Autodesk Fusion 360 part; units mm, degrees
(part 8 of 18)
  line L5222 (108.6972, -31.4557) -> (122.6972, -31.4557)
  line L5223 (122.6972, -45.4557) -> (108.6972, -45.4557)
  line L5224 (108.6972, -45.4557) -> (108.6972, -31.4557)
  line L5225 (89.6472, -26.4057) -> (89.6472, -12.4056)
  line L5226 (103.6472, -12.4056) -> (103.6472, -26.4057)
  line L5227 (103.6472, -26.4057) -> (89.6472, -26.4057)
  line L5228 (89.6472, -12.4056) -> (103.6472, -12.4056)
  line L5229 (89.6472, -31.4557) -> (103.6472, -31.4557)
  line L5230 (103.6472, -31.4557) -> (103.6472, -45.4557)
  line L5231 (103.6472, -45.4557) -> (89.6472, -45.4557)
  line L5232 (89.6472, -45.4557) -> (89.6472, -31.4557)
  line L5233 (89.6472, -69.5811) -> (103.6472, -69.5811)
  line L5234 (103.6472, -83.5812) -> (89.6472, -83.5812)
  line L5235 (103.6472, -69.5811) -> (103.6472, -83.5812)
  line L5236 (89.6472, -83.5812) -> (89.6472, -69.5811)
  line L5237 (89.6472, -64.5184) -> (89.6472, -50.5184)
  line L5238 (103.6472, -64.5184) -> (89.6472, -64.5184)
  line L5239 (89.6472, -50.5184) -> (103.6472, -50.5184)
  line L5240 (103.6472, -50.5184) -> (103.6472, -64.5184)
  line L5241 (184.8974, -83.5812) -> (184.8974, -69.5811)
  line L5242 (198.8974, -83.5812) -> (184.8974, -83.5812)
  line L5243 (198.8974, -69.5811) -> (198.8974, -83.5812)
  line L5244 (184.8974, -69.5811) -> (198.8974, -69.5811)
  line L5245 (184.8974, -12.4056) -> (198.8974, -12.4056)
  line L5246 (198.8974, -12.4056) -> (198.8974, -26.4057)
  line L5247 (198.8974, -26.4057) -> (184.8974, -26.4057)
  line L5248 (184.8974, -26.4057) -> (184.8974, -12.4056)
  line L5249 (84.5972, -83.5812) -> (70.5971, -83.5812)
  line L5250 (70.5971, -69.5811) -> (84.5972, -69.5811)
  line L5251 (70.5971, -83.5812) -> (70.5971, -69.5811)
  line L5252 (84.5972, -69.5811) -> (84.5972, -83.5812)
  line L5253 (70.5971, -31.4557) -> (84.5972, -31.4557)
  line L5254 (70.5971, -45.4557) -> (70.5971, -31.4557)
  line L5255 (84.5972, -31.4557) -> (84.5972, -45.4557)
  line L5256 (84.5972, -45.4557) -> (70.5971, -45.4557)
  line L5257 (70.5971, -12.4056) -> (84.5972, -12.4056)
  line L5258 (84.5972, -12.4056) -> (84.5972, -26.4057)
  line L5259 (70.5971, -26.4057) -> (70.5971, -12.4056)
  line L5260 (84.5972, -26.4057) -> (70.5971, -26.4057)
  line L5261 (70.5971, -50.5184) -> (84.5972, -50.5184)
  line L5262 (84.5972, -64.5184) -> (70.5971, -64.5184)
  line L5263 (70.5971, -64.5184) -> (70.5971, -50.5184)
  line L5264 (84.5972, -50.5184) -> (84.5972, -64.5184)
  line L5265 (65.5471, -83.5812) -> (51.5471, -83.5812)
  line L5266 (51.5471, -69.5811) -> (65.5471, -69.5811)
  line L5267 (51.5471, -83.5812) -> (51.5471, -69.5811)
  line L5268 (65.5471, -69.5811) -> (65.5471, -83.5812)
  line L5269 (65.5471, -50.5184) -> (65.5471, -64.5184)
  line L5270 (51.5471, -64.5184) -> (51.5471, -50.5184)
  line L5271 (65.5471, -64.5184) -> (51.5471, -64.5184)
  line L5272 (51.5471, -50.5184) -> (65.5471, -50.5184)
  line L5273 (51.5471, -45.4557) -> (51.5471, -31.4557)
  line L5274 (65.5471, -31.4557) -> (65.5471, -45.4557)
  line L5275 (51.5471, -31.4557) -> (65.5471, -31.4557)
  line L5276 (65.5471, -45.4557) -> (51.5471, -45.4557)
  line L5277 (46.4971, -64.5184) -> (32.4971, -64.5184)
  line L5278 (32.4971, -64.5184) -> (32.4971, -50.5184)
  line L5279 (32.4971, -50.5184) -> (46.4971, -50.5184)
  line L5280 (46.4971, -50.5184) -> (46.4971, -64.5184)
  line L5281 (32.4971, -69.5811) -> (46.4971, -69.5811)
  line L5282 (32.4971, -83.5812) -> (32.4971, -69.5811)
  line L5283 (46.4971, -83.5812) -> (32.4971, -83.5812)
  line L5284 (46.4971, -69.5811) -> (46.4971, -83.5812)
  line L5285 (13.447, -69.5811) -> (27.4471, -69.5811)
  line L5286 (27.4471, -83.5812) -> (13.447, -83.5812)
  line L5287 (27.4471, -69.5811) -> (27.4471, -83.5812)
  line L5288 (13.447, -83.5812) -> (13.447, -69.5811)
  line L5289 (-5.603, -69.5811) -> (8.397, -69.5811)
  line L5290 (8.397, -83.5812) -> (-5.603, -83.5812)
  line L5291 (8.397, -69.5811) -> (8.397, -83.5812)
  line L5292 (-5.603, -83.5812) -> (-5.603, -69.5811)
  line L5293 (65.5471, -12.4056) -> (65.5471, -26.4057)
  line L5294 (51.5471, -12.4056) -> (65.5471, -12.4056)
  line L5295 (51.5471, -26.4057) -> (51.5471, -12.4056)
  line L5296 (65.5471, -26.4057) -> (51.5471, -26.4057)
  line L5297 (32.4971, -31.4557) -> (46.4971, -31.4557)
  line L5298 (46.4971, -45.4557) -> (32.4971, -45.4557)
  line L5299 (32.4971, -45.4557) -> (32.4971, -31.4557)
  line L5300 (46.4971, -31.4557) -> (46.4971, -45.4557)
  line L5301 (46.4971, -12.4056) -> (46.4971, -26.4057)
  line L5302 (32.4971, -12.4056) -> (46.4971, -12.4056)
  line L5303 (32.4971, -26.4057) -> (32.4971, -12.4056)
  line L5304 (46.4971, -26.4057) -> (32.4971, -26.4057)
  line L5305 (13.447, -26.4057) -> (13.447, -12.4056)
  line L5306 (27.4471, -26.4057) -> (13.447, -26.4057)
  line L5307 (27.4471, -12.4056) -> (27.4471, -26.4057)
  line L5308 (13.447, -12.4056) -> (27.4471, -12.4056)
  line L5309 (13.447, -64.5184) -> (13.447, -50.5184)
  line L5310 (27.4471, -64.5184) -> (13.447, -64.5184)
  line L5311 (13.447, -50.5184) -> (27.4471, -50.5184)
  line L5312 (27.4471, -50.5184) -> (27.4471, -64.5184)
  line L5313 (13.447, -31.4557) -> (27.4471, -31.4557)
  line L5314 (27.4471, -45.4557) -> (13.447, -45.4557)
  line L5315 (27.4471, -31.4557) -> (27.4471, -45.4557)
  line L5316 (13.447, -45.4557) -> (13.447, -31.4557)
  line L5317 (8.397, -12.4056) -> (8.397, -26.4057)
  line L5318 (-5.603, -12.4056) -> (8.397, -12.4056)
  line L5319 (-5.603, -26.4057) -> (-5.603, -12.4056)
  line L5320 (8.397, -26.4057) -> (-5.603, -26.4057)
  line L5321 (8.397, -45.4557) -> (-5.603, -45.4557)
  line L5322 (8.397, -31.4557) -> (8.397, -45.4557)
  line L5323 (-5.603, -45.4557) -> (-5.603, -31.4557)
  line L5324 (-5.603, -31.4557) -> (8.397, -31.4557)
  line L5325 (-5.603, -50.5184) -> (8.397, -50.5184)
  line L5326 (8.397, -50.5184) -> (8.397, -64.5184)
  line L5327 (-5.603, -64.5184) -> (-5.603, -50.5184)
  line L5328 (8.397, -64.5184) -> (-5.603, -64.5184)
  line L5329 (217.9474, -50.5184) -> (217.9474, -64.5184)
  line L5330 (203.9474, -50.5184) -> (217.9474, -50.5184)
  line L5331 (217.9474, -64.5184) -> (203.9474, -64.5184)
  line L5332 (203.9474, -64.5184) -> (203.9474, -50.5184)
  line L5333 (203.9474, -31.4557) -> (217.9474, -31.4557)
  line L5334 (217.9474, -45.4557) -> (203.9474, -45.4557)
  line L5335 (203.9474, -45.4557) -> (203.9474, -31.4557)
  line L5336 (217.9474, -31.4557) -> (217.9474, -45.4557)
  line L5337 (217.9474, -12.4056) -> (217.9474, -26.4057)
  line L5338 (203.9474, -26.4057) -> (203.9474, -12.4056)
  line L5339 (217.9474, -26.4057) -> (203.9474, -26.4057)
  line L5340 (203.9474, -12.4056) -> (217.9474, -12.4056)
  line L5341 (203.9474, -69.5811) -> (217.9474, -69.5811)
  line L5342 (203.9474, -83.5812) -> (203.9474, -69.5811)
  line L5343 (217.9474, -83.5812) -> (203.9474, -83.5812)
  line L5344 (217.9474, -69.5811) -> (217.9474, -83.5812)
  line L5345 (184.8974, -45.4557) -> (184.8974, -31.4557)
  line L5346 (198.8974, -31.4557) -> (198.8974, -45.4557)
  line L5347 (184.8974, -31.4557) -> (198.8974, -31.4557)
  line L5348 (198.8974, -45.4557) -> (184.8974, -45.4557)
  line L5349 (177.1674, -3.048) -> (172.3373, -3.048)
  line L5350 (177.1674, -5.588) -> (177.1674, -3.048)
  line L5351 (177.1674, -5.588) -> (172.3373, -5.588)
  line L5352 (172.3373, -5.588) -> (172.3373, -3.048)
  line L5353 (188.5494, -4.29) -> (189.1994, -4.29)
  line L5354 (188.5494, -5.49) -> (188.5494, -4.29)
  line L5355 (189.1994, -4.29) -> (189.1994, -5.49)
  line L5356 (189.1994, -5.49) -> (188.5494, -5.49)
  line L5357 (188.3993, -5.49) -> (187.7493, -5.49)
  line L5358 (188.3993, -4.29) -> (188.3993, -5.49)
  line L5359 (187.7493, -4.29) -> (188.3993, -4.29)
  line L5360 (187.7493, -5.49) -> (187.7493, -4.29)
  line L5361 (187.6243, -4.29) -> (187.6243, -5.49)
  line L5362 (187.6243, -5.49) -> (187.2243, -5.49)
  line L5363 (187.2243, -4.29) -> (187.6243, -4.29)
  line L5364 (187.2243, -5.49) -> (187.2243, -4.29)
  line L5365 (187.1242, -5.49) -> (186.7242, -5.49)
  line L5366 (186.7242, -4.29) -> (187.1242, -4.29)
  line L5367 (187.1242, -4.29) -> (187.1242, -5.49)
  line L5368 (186.7242, -5.49) -> (186.7242, -4.29)
  line L5369 (186.2243, -4.29) -> (186.6243, -4.29)
  line L5370 (186.2243, -5.49) -> (186.2243, -4.29)
  line L5371 (186.6243, -5.49) -> (186.2243, -5.49)
  line L5372 (186.6243, -4.29) -> (186.6243, -5.49)
  line L5373 (185.7244, -5.49) -> (185.7244, -4.29)
  line L5374 (186.1244, -4.29) -> (186.1244, -5.49)
  line L5375 (186.1244, -5.49) -> (185.7244, -5.49)
  line L5376 (185.7244, -4.29) -> (186.1244, -4.29)
  line L5377 (185.6243, -5.49) -> (185.2243, -5.49)
  line L5378 (185.2243, -5.49) -> (185.2243, -4.29)
  line L5379 (185.2243, -4.29) -> (185.6243, -4.29)
  line L5380 (185.6243, -4.29) -> (185.6243, -5.49)
  line L5381 (185.1244, -4.29) -> (185.1244, -5.49)
  line L5382 (185.1244, -5.49) -> (184.7244, -5.49)
  line L5383 (184.7244, -4.29) -> (185.1244, -4.29)
  line L5384 (184.7244, -5.49) -> (184.7244, -4.29)
  line L5385 (184.6243, -5.49) -> (184.2243, -5.49)
  line L5386 (184.2243, -4.29) -> (184.6243, -4.29)
  line L5387 (184.6243, -4.29) -> (184.6243, -5.49)
  line L5388 (184.2243, -5.49) -> (184.2243, -4.29)
  line L5389 (184.1242, -5.49) -> (183.7242, -5.49)
  line L5390 (183.7242, -5.49) -> (183.7242, -4.29)
  line L5391 (183.7242, -4.29) -> (184.1242, -4.29)
  line L5392 (184.1242, -4.29) -> (184.1242, -5.49)
  line L5393 (183.5992, -5.49) -> (182.9492, -5.49)
  line L5394 (183.5992, -4.29) -> (183.5992, -5.49)
  line L5395 (182.9492, -4.29) -> (183.5992, -4.29)
  line L5396 (182.9492, -5.49) -> (182.9492, -4.29)
  line L5397 (182.7994, -5.49) -> (182.1493, -5.49)
  line L5398 (182.7994, -4.29) -> (182.7994, -5.49)
  line L5399 (182.1493, -4.29) -> (182.7994, -4.29)
  line L5400 (182.1493, -5.49) -> (182.1493, -4.29)
  line L5401 (189.4747, -3.4901) -> (189.6943, -3.2705)
  line L5402 (190.2943, -3.2705) -> (190.5139, -3.4901)
  line L5403 (190.2943, -5.4097) -> (189.9943, -5.4901)
  line L5404 (190.5139, -3.4901) -> (190.5943, -3.7901)
  line L5405 (189.6943, -5.4097) -> (189.4747, -5.1901)
  line L5406 (189.6943, -3.2705) -> (189.9943, -3.1901)
  line L5407 (190.5139, -5.1901) -> (190.2943, -5.4097)
  line L5408 (189.3943, -3.7901) -> (189.4747, -3.4901)
  line L5409 (189.3943, -4.8901) -> (189.3943, -3.7901)
  line L5410 (189.9943, -5.4901) -> (189.6943, -5.4097)
  line L5411 (189.4747, -5.1901) -> (189.3943, -4.8901)
  line L5412 (189.9943, -3.1901) -> (190.2943, -3.2705)
  line L5413 (190.5943, -4.8901) -> (190.5139, -5.1901)
  line L5414 (190.5943, -3.7901) -> (190.5943, -4.8901)
  line L5415 (181.6545, -5.4097) -> (181.3545, -5.4901)
  line L5416 (181.0545, -5.4097) -> (180.8348, -5.1901)
  line L5417 (180.7544, -3.7901) -> (180.8348, -3.4901)
  line L5418 (181.8741, -3.4901) -> (181.9545, -3.7901)
  line L5419 (180.8348, -5.1901) -> (180.7544, -4.8901)
  line L5420 (181.9545, -3.7901) -> (181.9545, -4.8901)
  line L5421 (181.9545, -4.8901) -> (181.8741, -5.1901)
  line L5422 (181.8741, -5.1901) -> (181.6545, -5.4097)
  line L5423 (180.8348, -3.4901) -> (181.0545, -3.2705)
  line L5424 (181.3545, -3.1901) -> (181.6545, -3.2705)
  line L5425 (181.0545, -3.2705) -> (181.3545, -3.1901)
  line L5426 (180.7544, -4.8901) -> (180.7544, -3.7901)
  line L5427 (181.3545, -5.4901) -> (181.0545, -5.4097)
  line L5428 (181.6545, -3.2705) -> (181.8741, -3.4901)
  line L5429 (189.3943, 0.21) -> (189.4747, 0.51)
  line L5430 (189.3943, -0.59) -> (189.3943, 0.21)
  line L5431 (190.5943, 0.21) -> (190.5943, -0.59)
  line L5432 (190.5139, -0.89) -> (190.2943, -1.1096)
  line L5433 (190.5139, 0.51) -> (190.5943, 0.21)
  line L5434 (189.4747, 0.51) -> (189.6943, 0.7297)
  line L5435 (189.6943, 0.7297) -> (189.9943, 0.81)
  line L5436 (190.5943, -0.59) -> (190.5139, -0.89)
  line L5437 (189.9943, -1.19) -> (189.6943, -1.1096)
  line L5438 (189.9943, 0.81) -> (190.2943, 0.7297)
  line L5439 (190.2943, 0.7297) -> (190.5139, 0.51)
  line L5440 (190.2943, -1.1096) -> (189.9943, -1.19)
  line L5441 (189.6943, -1.1096) -> (189.4747, -0.89)
  line L5442 (189.4747, -0.89) -> (189.3943, -0.59)
  line L5443 (181.0545, 0.7297) -> (181.3545, 0.81)
  line L5444 (181.3545, 0.81) -> (181.6545, 0.7297)
  line L5445 (181.8741, 0.51) -> (181.9545, 0.21)
  line L5446 (180.8348, 0.51) -> (181.0545, 0.7297)
  line L5447 (181.0545, -1.1096) -> (180.8348, -0.89)
  line L5448 (180.8348, -0.89) -> (180.7544, -0.59)
  line L5449 (181.8741, -0.89) -> (181.6545, -1.1096)
  line L5450 (181.9545, 0.21) -> (181.9545, -0.59)
  line L5451 (181.9545, -0.59) -> (181.8741, -0.89)
  line L5452 (180.7544, -0.59) -> (180.7544, 0.21)
  line L5453 (181.6545, -1.1096) -> (181.3545, -1.19)
  line L5454 (180.7544, 0.21) -> (180.8348, 0.51)
  line L5455 (181.6545, 0.7297) -> (181.8741, 0.51)
  line L5456 (181.3545, -1.19) -> (181.0545, -1.1096)
  line L5457 (200.3611, -1.4222) -> (200.3611, -2.3878)
  line L5458 (200.3611, -2.3878) -> (199.453, -2.3878)
  line L5459 (199.453, -1.4222) -> (200.3611, -1.4222)
  line L5460 (199.453, -2.3878) -> (199.453, -1.4222)
  line L5461 (200.9597, -1.4222) -> (201.8678, -1.4222)
  line L5462 (201.8678, -1.4222) -> (201.8678, -2.3878)
  line L5463 (201.8678, -2.3878) -> (200.9597, -2.3878)
  line L5464 (200.9597, -2.3878) -> (200.9597, -1.4222)
  line L5465 (207.2836, -6.3137) -> (207.2836, -6.0121)
  line L5466 (207.2836, -6.0121) -> (208.0502, -6.0121)
  line L5467 (208.0502, -6.0121) -> (208.0502, -6.3137)
  line L5468 (208.0502, -6.3137) -> (207.2836, -6.3137)
  line L5469 (208.0502, -6.4122) -> (208.0502, -6.7138)
  line L5470 (207.2836, -6.7138) -> (207.2836, -6.4122)
  line L5471 (208.0502, -6.7138) -> (207.2836, -6.7138)
  line L5472 (207.2836, -6.4122) -> (208.0502, -6.4122)
  line L5473 (208.0502, -7.1138) -> (207.2836, -7.1138)
  line L5474 (207.2836, -7.1138) -> (207.2836, -6.8122)
  line L5475 (207.2836, -6.8122) -> (208.0502, -6.8122)
  line L5476 (208.0502, -6.8122) -> (208.0502, -7.1138)
  line L5477 (208.0502, -7.212) -> (208.0502, -7.5136)
  line L5478 (207.2836, -7.5136) -> (207.2836, -7.212)
  line L5479 (208.0502, -7.5136) -> (207.2836, -7.5136)
  line L5480 (207.2836, -7.212) -> (208.0502, -7.212)
  line L5481 (207.2836, -7.6121) -> (208.0502, -7.6121)
  line L5482 (208.0502, -7.6121) -> (208.0502, -7.9137)
  line L5483 (208.0502, -7.9137) -> (207.2836, -7.9137)
  line L5484 (207.2836, -7.9137) -> (207.2836, -7.6121)
  line L5485 (207.2836, -8.3137) -> (207.2836, -8.0121)
  line L5486 (208.0502, -8.3137) -> (207.2836, -8.3137)
  line L5487 (207.2836, -8.0121) -> (208.0502, -8.0121)
  line L5488 (208.0502, -8.0121) -> (208.0502, -8.3137)
  line L5489 (208.0502, -8.7138) -> (207.2836, -8.7138)
  line L5490 (208.0502, -8.4122) -> (208.0502, -8.7138)
  line L5491 (207.2836, -8.4122) -> (208.0502, -8.4122)
  line L5492 (207.2836, -8.7138) -> (207.2836, -8.4122)
  line L5493 (208.0502, -8.8122) -> (208.0502, -9.1138)
  line L5494 (208.0502, -9.1138) -> (207.2836, -9.1138)
  line L5495 (207.2836, -8.8122) -> (208.0502, -8.8122)
  line L5496 (207.2836, -9.1138) -> (207.2836, -8.8122)
  line L5497 (208.0502, -9.5136) -> (207.2836, -9.5136)
  line L5498 (208.0502, -9.212) -> (208.0502, -9.5136)
  line L5499 (207.2836, -9.5136) -> (207.2836, -9.212)
  line L5500 (207.2836, -9.212) -> (208.0502, -9.212)
  line L5501 (208.0502, -9.9137) -> (207.2836, -9.9137)
  line L5502 (208.0502, -9.6121) -> (208.0502, -9.9137)
  line L5503 (207.2836, -9.9137) -> (207.2836, -9.6121)
  line L5504 (207.2836, -9.6121) -> (208.0502, -9.6121)
  line L5505 (207.2836, -10.3137) -> (207.2836, -10.0121)
  line L5506 (208.0502, -10.0121) -> (208.0502, -10.3137)
  line L5507 (208.0502, -10.3137) -> (207.2836, -10.3137)
  line L5508 (207.2836, -10.0121) -> (208.0502, -10.0121)
  line L5509 (208.0502, -10.7138) -> (207.2836, -10.7138)
  line L5510 (207.2836, -10.4122) -> (208.0502, -10.4122)
  line L5511 (207.2836, -10.7138) -> (207.2836, -10.4122)
  line L5512 (208.0502, -10.4122) -> (208.0502, -10.7138)
  line L5513 (207.2836, -11.1138) -> (207.2836, -10.8122)
  line L5514 (208.0502, -11.1138) -> (207.2836, -11.1138)
  line L5515 (208.0502, -10.8122) -> (208.0502, -11.1138)
  line L5516 (207.2836, -10.8122) -> (208.0502, -10.8122)
  line L5517 (208.0502, -11.212) -> (208.0502, -11.5136)
  line L5518 (207.2836, -11.5136) -> (207.2836, -11.212)
  line L5519 (207.2836, -11.212) -> (208.0502, -11.212)
  line L5520 (208.0502, -11.5136) -> (207.2836, -11.5136)
  line L5521 (208.6254, -11.7873) -> (208.6254, -12.5539)
  line L5522 (208.6254, -12.5539) -> (208.3238, -12.5539)
  line L5523 (208.3238, -12.5539) -> (208.3238, -11.7873)
  line L5524 (208.3238, -11.7873) -> (208.6254, -11.7873)
  line L5525 (209.0252, -11.7873) -> (209.0252, -12.5539)
  line L5526 (208.7236, -11.7873) -> (209.0252, -11.7873)
  line L5527 (209.0252, -12.5539) -> (208.7236, -12.5539)
  line L5528 (208.7236, -12.5539) -> (208.7236, -11.7873)
  line L5529 (209.4252, -11.7873) -> (209.4252, -12.5539)
  line L5530 (209.1236, -12.5539) -> (209.1236, -11.7873)
  line L5531 (209.4252, -12.5539) -> (209.1236, -12.5539)
  line L5532 (209.1236, -11.7873) -> (209.4252, -11.7873)
  line L5533 (209.5237, -11.7873) -> (209.8253, -11.7873)
  line L5534 (209.8253, -12.5539) -> (209.5237, -12.5539)
  line L5535 (209.5237, -12.5539) -> (209.5237, -11.7873)
  line L5536 (209.8253, -11.7873) -> (209.8253, -12.5539)
  line L5537 (209.9237, -11.7873) -> (210.2253, -11.7873)
  line L5538 (210.2253, -11.7873) -> (210.2253, -12.5539)
  line L5539 (210.2253, -12.5539) -> (209.9237, -12.5539)
  line L5540 (209.9237, -12.5539) -> (209.9237, -11.7873)
  line L5541 (210.3238, -11.7873) -> (210.6254, -11.7873)
  line L5542 (210.6254, -12.5539) -> (210.3238, -12.5539)
  line L5543 (210.6254, -11.7873) -> (210.6254, -12.5539)
  line L5544 (210.3238, -12.5539) -> (210.3238, -11.7873)
  line L5545 (211.0252, -12.5539) -> (210.7236, -12.5539)
  line L5546 (211.0252, -11.7873) -> (211.0252, -12.5539)
  line L5547 (210.7236, -11.7873) -> (211.0252, -11.7873)
  line L5548 (210.7236, -12.5539) -> (210.7236, -11.7873)
  line L5549 (211.1236, -12.5539) -> (211.1236, -11.7873)
  line L5550 (211.4252, -12.5539) -> (211.1236, -12.5539)
  line L5551 (211.1236, -11.7873) -> (211.4252, -11.7873)
  line L5552 (211.4252, -11.7873) -> (211.4252, -12.5539)
  line L5553 (211.5237, -11.7873) -> (211.8253, -11.7873)
  line L5554 (211.5237, -12.5539) -> (211.5237, -11.7873)
  line L5555 (211.8253, -12.5539) -> (211.5237, -12.5539)
  line L5556 (211.8253, -11.7873) -> (211.8253, -12.5539)
  line L5557 (211.9237, -12.5539) -> (211.9237, -11.7873)
  line L5558 (212.2253, -12.5539) -> (211.9237, -12.5539)
  line L5559 (212.2253, -11.7873) -> (212.2253, -12.5539)
  line L5560 (211.9237, -11.7873) -> (212.2253, -11.7873)
  line L5561 (212.3238, -12.5539) -> (212.3238, -11.7873)
  line L5562 (212.3238, -11.7873) -> (212.6254, -11.7873)
  line L5563 (212.6254, -12.5539) -> (212.3238, -12.5539)
  line L5564 (212.6254, -11.7873) -> (212.6254, -12.5539)
  line L5565 (213.0252, -11.7873) -> (213.0252, -12.5539)
  line L5566 (212.7236, -12.5539) -> (212.7236, -11.7873)
  line L5567 (213.0252, -12.5539) -> (212.7236, -12.5539)
  line L5568 (212.7236, -11.7873) -> (213.0252, -11.7873)
  line L5569 (213.1236, -12.5539) -> (213.1236, -11.7873)
  line L5570 (213.4252, -11.7873) -> (213.4252, -12.5539)
  line L5571 (213.4252, -12.5539) -> (213.1236, -12.5539)
  line L5572 (213.1236, -11.7873) -> (213.4252, -11.7873)
  line L5573 (213.5237, -12.5539) -> (213.5237, -11.7873)
  line L5574 (213.8253, -12.5539) -> (213.5237, -12.5539)
  line L5575 (213.8253, -11.7873) -> (213.8253, -12.5539)
  line L5576 (213.5237, -11.7873) -> (213.8253, -11.7873)
  line L5577 (214.8653, -11.212) -> (214.8653, -11.5136)
  line L5578 (214.0987, -11.212) -> (214.8653, -11.212)
  line L5579 (214.8653, -11.5136) -> (214.0987, -11.5136)
  line L5580 (214.0987, -11.5136) -> (214.0987, -11.212)
  line L5581 (214.0987, -11.1138) -> (214.0987, -10.8122)
  line L5582 (214.8653, -11.1138) -> (214.0987, -11.1138)
  line L5583 (214.0987, -10.8122) -> (214.8653, -10.8122)
  line L5584 (214.8653, -10.8122) -> (214.8653, -11.1138)
  line L5585 (214.0987, -10.7138) -> (214.0987, -10.4122)
  line L5586 (214.0987, -10.4122) -> (214.8653, -10.4122)
  line L5587 (214.8653, -10.4122) -> (214.8653, -10.7138)
  line L5588 (214.8653, -10.7138) -> (214.0987, -10.7138)
  line L5589 (214.0987, -10.0121) -> (214.8653, -10.0121)
  line L5590 (214.8653, -10.0121) -> (214.8653, -10.3137)
  line L5591 (214.8653, -10.3137) -> (214.0987, -10.3137)
  line L5592 (214.0987, -10.3137) -> (214.0987, -10.0121)
  line L5593 (214.8653, -9.6121) -> (214.8653, -9.9137)
  line L5594 (214.0987, -9.6121) -> (214.8653, -9.6121)
  line L5595 (214.8653, -9.9137) -> (214.0987, -9.9137)
  line L5596 (214.0987, -9.9137) -> (214.0987, -9.6121)
  line L5597 (214.0987, -9.212) -> (214.8653, -9.212)
  line L5598 (214.8653, -9.212) -> (214.8653, -9.5136)
  line L5599 (214.0987, -9.5136) -> (214.0987, -9.212)
  line L5600 (214.8653, -9.5136) -> (214.0987, -9.5136)
  line L5601 (214.0987, -9.1138) -> (214.0987, -8.8122)
  line L5602 (214.0987, -8.8122) -> (214.8653, -8.8122)
  line L5603 (214.8653, -9.1138) -> (214.0987, -9.1138)
  line L5604 (214.8653, -8.8122) -> (214.8653, -9.1138)
  line L5605 (214.0987, -8.7138) -> (214.0987, -8.4122)
  line L5606 (214.8653, -8.4122) -> (214.8653, -8.7138)
  line L5607 (214.0987, -8.4122) -> (214.8653, -8.4122)
  line L5608 (214.8653, -8.7138) -> (214.0987, -8.7138)
  line L5609 (214.8653, -8.0121) -> (214.8653, -8.3137)
  line L5610 (214.0987, -8.3137) -> (214.0987, -8.0121)
  line L5611 (214.0987, -8.0121) -> (214.8653, -8.0121)
  line L5612 (214.8653, -8.3137) -> (214.0987, -8.3137)
  line L5613 (214.8653, -7.9137) -> (214.0987, -7.9137)
  line L5614 (214.0987, -7.9137) -> (214.0987, -7.6121)
  line L5615 (214.0987, -7.6121) -> (214.8653, -7.6121)
  line L5616 (214.8653, -7.6121) -> (214.8653, -7.9137)
  line L5617 (214.8653, -7.212) -> (214.8653, -7.5136)
  line L5618 (214.0987, -7.212) -> (214.8653, -7.212)
  line L5619 (214.0987, -7.5136) -> (214.0987, -7.212)
  line L5620 (214.8653, -7.5136) -> (214.0987, -7.5136)
  line L5621 (214.8653, -7.1138) -> (214.0987, -7.1138)
  line L5622 (214.0987, -7.1138) -> (214.0987, -6.8122)
  line L5623 (214.8653, -6.8122) -> (214.8653, -7.1138)
  line L5624 (214.0987, -6.8122) -> (214.8653, -6.8122)
  line L5625 (214.8653, -6.4122) -> (214.8653, -6.7138)
  line L5626 (214.0987, -6.7138) -> (214.0987, -6.4122)
  line L5627 (214.0987, -6.4122) -> (214.8653, -6.4122)
  line L5628 (214.8653, -6.7138) -> (214.0987, -6.7138)
  line L5629 (214.8653, -6.0121) -> (214.8653, -6.3137)
  line L5630 (214.8653, -6.3137) -> (214.0987, -6.3137)
  line L5631 (214.0987, -6.3137) -> (214.0987, -6.0121)
  line L5632 (214.0987, -6.0121) -> (214.8653, -6.0121)
  line L5633 (213.8253, -5.7388) -> (213.5237, -5.7388)
  line L5634 (213.5237, -4.9722) -> (213.8253, -4.9722)
  line L5635 (213.8253, -4.9722) -> (213.8253, -5.7388)
  line L5636 (213.5237, -5.7388) -> (213.5237, -4.9722)
  line L5637 (213.1236, -4.9722) -> (213.4252, -4.9722)
  line L5638 (213.1236, -5.7388) -> (213.1236, -4.9722)
  line L5639 (213.4252, -4.9722) -> (213.4252, -5.7388)
  line L5640 (213.4252, -5.7388) -> (213.1236, -5.7388)
  line L5641 (212.7236, -5.7388) -> (212.7236, -4.9722)
  line L5642 (212.7236, -4.9722) -> (213.0252, -4.9722)
  line L5643 (213.0252, -5.7388) -> (212.7236, -5.7388)
  line L5644 (213.0252, -4.9722) -> (213.0252, -5.7388)
  line L5645 (212.6254, -4.9722) -> (212.6254, -5.7388)
  line L5646 (212.3238, -4.9722) -> (212.6254, -4.9722)
  line L5647 (212.6254, -5.7388) -> (212.3238, -5.7388)
  line L5648 (212.3238, -5.7388) -> (212.3238, -4.9722)
  line L5649 (212.2253, -5.7388) -> (211.9237, -5.7388)
  line L5650 (211.9237, -4.9722) -> (212.2253, -4.9722)
  line L5651 (212.2253, -4.9722) -> (212.2253, -5.7388)
  line L5652 (211.9237, -5.7388) -> (211.9237, -4.9722)
  line L5653 (211.5237, -5.7388) -> (211.5237, -4.9722)
  line L5654 (211.5237, -4.9722) -> (211.8253, -4.9722)
  line L5655 (211.8253, -5.7388) -> (211.5237, -5.7388)
  line L5656 (211.8253, -4.9722) -> (211.8253, -5.7388)
  line L5657 (211.4252, -4.9722) -> (211.4252, -5.7388)
  line L5658 (211.1236, -5.7388) -> (211.1236, -4.9722)
  line L5659 (211.1236, -4.9722) -> (211.4252, -4.9722)
  line L5660 (211.4252, -5.7388) -> (211.1236, -5.7388)
  line L5661 (211.0252, -4.9722) -> (211.0252, -5.7388)
  line L5662 (210.7236, -4.9722) -> (211.0252, -4.9722)
  line L5663 (210.7236, -5.7388) -> (210.7236, -4.9722)
  line L5664 (211.0252, -5.7388) -> (210.7236, -5.7388)
  line L5665 (210.6254, -4.9722) -> (210.6254, -5.7388)
  line L5666 (210.3238, -4.9722) -> (210.6254, -4.9722)
  line L5667 (210.6254, -5.7388) -> (210.3238, -5.7388)
  line L5668 (210.3238, -5.7388) -> (210.3238, -4.9722)
  line L5669 (209.9237, -5.7388) -> (209.9237, -4.9722)
  line L5670 (210.2253, -4.9722) -> (210.2253, -5.7388)
  line L5671 (209.9237, -4.9722) -> (210.2253, -4.9722)
  line L5672 (210.2253, -5.7388) -> (209.9237, -5.7388)
  line L5673 (209.8253, -5.7388) -> (209.5237, -5.7388)
  line L5674 (209.5237, -5.7388) -> (209.5237, -4.9722)
  line L5675 (209.5237, -4.9722) -> (209.8253, -4.9722)
  line L5676 (209.8253, -4.9722) -> (209.8253, -5.7388)
  line L5677 (209.1236, -5.7388) -> (209.1236, -4.9722)
  line L5678 (209.4252, -5.7388) -> (209.1236, -5.7388)
  line L5679 (209.4252, -4.9722) -> (209.4252, -5.7388)
  line L5680 (209.1236, -4.9722) -> (209.4252, -4.9722)
  line L5681 (209.0252, -4.9722) -> (209.0252, -5.7388)
  line L5682 (208.7236, -5.7388) -> (208.7236, -4.9722)
  line L5683 (208.7236, -4.9722) -> (209.0252, -4.9722)
  line L5684 (209.0252, -5.7388) -> (208.7236, -5.7388)
  line L5685 (208.6254, -5.7388) -> (208.3238, -5.7388)
  line L5686 (208.6254, -4.9722) -> (208.6254, -5.7388)
  line L5687 (208.3238, -5.7388) -> (208.3238, -4.9722)
  line L5688 (208.3238, -4.9722) -> (208.6254, -4.9722)
  line L5689 (209.0237, -10.8137) -> (209.0237, -6.7121)
  line L5690 (213.1253, -10.8137) -> (209.0237, -10.8137)
  line L5691 (209.0237, -6.7121) -> (213.1253, -6.7121)
  line L5692 (213.1253, -6.7121) -> (213.1253, -10.8137)
  line L5693 (188.9138, -6.2482) -> (188.9138, -7.2138)
  line L5694 (188.0057, -7.2138) -> (188.0057, -6.2482)
  line L5695 (188.9138, -7.2138) -> (188.0057, -7.2138)
  line L5696 (188.0057, -6.2482) -> (188.9138, -6.2482)
  line L5697 (187.407, -6.2482) -> (187.407, -7.2138)
  line L5698 (186.499, -6.2482) -> (187.407, -6.2482)
  line L5699 (187.407, -7.2138) -> (186.499, -7.2138)
  line L5700 (186.499, -7.2138) -> (186.499, -6.2482)
  line L5701 (182.835, -6.2482) -> (182.835, -7.2138)
  line L5702 (181.927, -6.2482) -> (182.835, -6.2482)
  line L5703 (181.927, -7.2138) -> (181.927, -6.2482)
  line L5704 (182.835, -7.2138) -> (181.927, -7.2138)
  line L5705 (184.3418, -7.2138) -> (183.4337, -7.2138)
  line L5706 (184.3418, -6.2482) -> (184.3418, -7.2138)
  line L5707 (183.4337, -6.2482) -> (184.3418, -6.2482)
  line L5708 (183.4337, -7.2138) -> (183.4337, -6.2482)
  line L5709 (211.8344, -3.0849) -> (213.2364, -3.0849)
  line L5710 (211.8344, -3.4869) -> (211.8344, -3.0849)
  line L5711 (213.2364, -3.0849) -> (213.2364, -3.4869)
  line L5712 (213.2364, -3.4869) -> (211.8344, -3.4869)
  line L5713 (213.2364, -2.585) -> (213.2364, -2.987)
  line L5714 (211.8344, -2.585) -> (213.2364, -2.585)
  line L5715 (213.2364, -2.987) -> (211.8344, -2.987)
  line L5716 (211.8344, -2.987) -> (211.8344, -2.585)
  line L5717 (211.8344, -2.0851) -> (213.2364, -2.0851)
  line L5718 (211.8344, -2.4871) -> (211.8344, -2.0851)
  line L5719 (213.2364, -2.0851) -> (213.2364, -2.4871)
  line L5720 (213.2364, -2.4871) -> (211.8344, -2.4871)
  line L5721 (213.2364, -1.585) -> (213.2364, -1.987)
  line L5722 (211.8344, -1.585) -> (213.2364, -1.585)
  line L5723 (213.2364, -1.987) -> (211.8344, -1.987)
  line L5724 (211.8344, -1.987) -> (211.8344, -1.585)
  line L5725 (213.2364, -1.4869) -> (211.8344, -1.4869)
  line L5726 (211.8344, -1.4869) -> (211.8344, -1.0849)
  line L5727 (213.2364, -1.0849) -> (213.2364, -1.4869)
  line L5728 (211.8344, -1.0849) -> (213.2364, -1.0849)
  line L5729 (207.1344, -1.0851) -> (208.5364, -1.0851)
  line L5730 (207.1344, -1.4871) -> (207.1344, -1.0851)
  line L5731 (208.5364, -1.0851) -> (208.5364, -1.4871)
  line L5732 (208.5364, -1.4871) -> (207.1344, -1.4871)
  line L5733 (208.5364, -1.585) -> (208.5364, -1.987)
  line L5734 (207.1344, -1.987) -> (207.1344, -1.585)
  line L5735 (208.5364, -1.987) -> (207.1344, -1.987)
  line L5736 (207.1344, -1.585) -> (208.5364, -1.585)
  line L5737 (207.1344, -2.4869) -> (207.1344, -2.0849)
  line L5738 (207.1344, -2.0849) -> (208.5364, -2.0849)
  line L5739 (208.5364, -2.4869) -> (207.1344, -2.4869)
  line L5740 (208.5364, -2.0849) -> (208.5364, -2.4869)
  line L5741 (208.5364, -2.987) -> (207.1344, -2.987)
  line L5742 (207.1344, -2.987) -> (207.1344, -2.585)
  line L5743 (208.5364, -2.585) -> (208.5364, -2.987)
  line L5744 (207.1344, -2.585) -> (208.5364, -2.585)
  line L5745 (207.1344, -3.4871) -> (207.1344, -3.0851)
  line L5746 (208.5364, -3.4871) -> (207.1344, -3.4871)
  line L5747 (208.5364, -3.0851) -> (208.5364, -3.4871)
  line L5748 (207.1344, -3.0851) -> (208.5364, -3.0851)
  line L5749 (139.186, -76.3898) -> (139.186, -77.3314)
  line L5750 (139.186, -77.3314) -> (138.1744, -77.3314)
  line L5751 (138.1744, -76.3898) -> (139.186, -76.3898)
  line L5752 (138.1744, -77.3314) -> (138.1744, -76.3898)
  line L5753 (142.4962, -76.3898) -> (142.4962, -77.3314)
  line L5754 (141.4845, -77.3314) -> (141.4845, -76.3898)
  line L5755 (142.4962, -77.3314) -> (141.4845, -77.3314)
  line L5756 (141.4845, -76.3898) -> (142.4962, -76.3898)
  line L5757 (138.1744, -20.1558) -> (138.1744, -19.2142)
  line L5758 (138.1744, -19.2142) -> (139.186, -19.2142)
  line L5759 (139.186, -20.1558) -> (138.1744, -20.1558)
  line L5760 (139.186, -19.2142) -> (139.186, -20.1558)
  line L5761 (142.4962, -19.2142) -> (142.4962, -20.1558)
  line L5762 (141.4845, -20.1558) -> (141.4845, -19.2142)
  line L5763 (141.4845, -19.2142) -> (142.4962, -19.2142)
  line L5764 (142.4962, -20.1558) -> (141.4845, -20.1558)
  line L5765 (139.186, -39.2059) -> (138.1744, -39.2059)
  line L5766 (139.186, -38.2643) -> (139.186, -39.2059)
  line L5767 (138.1744, -39.2059) -> (138.1744, -38.2643)
  line L5768 (138.1744, -38.2643) -> (139.186, -38.2643)
  line L5769 (142.4962, -38.2643) -> (142.4962, -39.2059)
  line L5770 (141.4845, -38.2643) -> (142.4962, -38.2643)
  line L5771 (142.4962, -39.2059) -> (141.4845, -39.2059)
  line L5772 (141.4845, -39.2059) -> (141.4845, -38.2643)
  line L5773 (139.186, -57.327) -> (139.186, -58.2686)
  line L5774 (138.1744, -57.327) -> (139.186, -57.327)
  line L5775 (138.1744, -58.2686) -> (138.1744, -57.327)
  line L5776 (139.186, -58.2686) -> (138.1744, -58.2686)
  line L5777 (141.4845, -58.2686) -> (141.4845, -57.327)
  line L5778 (142.4962, -57.327) -> (142.4962, -58.2686)
  line L5779 (141.4845, -57.327) -> (142.4962, -57.327)
  line L5780 (142.4962, -58.2686) -> (141.4845, -58.2686)
  line L5781 (158.2361, -19.2142) -> (158.2361, -20.1558)
  line L5782 (158.2361, -20.1558) -> (157.2244, -20.1558)
  line L5783 (157.2244, -19.2142) -> (158.2361, -19.2142)
  line L5784 (157.2244, -20.1558) -> (157.2244, -19.2142)
  line L5785 (161.5462, -19.2142) -> (161.5462, -20.1558)
  line L5786 (160.5346, -19.2142) -> (161.5462, -19.2142)
  line L5787 (161.5462, -20.1558) -> (160.5346, -20.1558)
  line L5788 (160.5346, -20.1558) -> (160.5346, -19.2142)
  line L5789 (158.2361, -76.3898) -> (158.2361, -77.3314)
  line L5790 (157.2244, -76.3898) -> (158.2361, -76.3898)
  line L5791 (158.2361, -77.3314) -> (157.2244, -77.3314)
  line L5792 (157.2244, -77.3314) -> (157.2244, -76.3898)
  line L5793 (160.5346, -77.3314) -> (160.5346, -76.3898)
  line L5794 (161.5462, -77.3314) -> (160.5346, -77.3314)
  line L5795 (161.5462, -76.3898) -> (161.5462, -77.3314)
  line L5796 (160.5346, -76.3898) -> (161.5462, -76.3898)
  line L5797 (158.2361, -58.2686) -> (157.2244, -58.2686)
  line L5798 (157.2244, -57.327) -> (158.2361, -57.327)
  line L5799 (157.2244, -58.2686) -> (157.2244, -57.327)
  line L5800 (158.2361, -57.327) -> (158.2361, -58.2686)
  line L5801 (161.5462, -57.327) -> (161.5462, -58.2686)
  line L5802 (160.5346, -58.2686) -> (160.5346, -57.327)
  line L5803 (161.5462, -58.2686) -> (160.5346, -58.2686)
  line L5804 (160.5346, -57.327) -> (161.5462, -57.327)
  line L5805 (157.2244, -39.2059) -> (157.2244, -38.2643)
  line L5806 (158.2361, -39.2059) -> (157.2244, -39.2059)
  line L5807 (157.2244, -38.2643) -> (158.2361, -38.2643)
  line L5808 (158.2361, -38.2643) -> (158.2361, -39.2059)
  line L5809 (160.5346, -39.2059) -> (160.5346, -38.2643)
  line L5810 (161.5462, -39.2059) -> (160.5346, -39.2059)
  line L5811 (161.5462, -38.2643) -> (161.5462, -39.2059)
  line L5812 (160.5346, -38.2643) -> (161.5462, -38.2643)
  line L5813 (176.2745, -20.1558) -> (176.2745, -19.2142)
  line L5814 (177.2861, -20.1558) -> (176.2745, -20.1558)
  line L5815 (176.2745, -19.2142) -> (177.2861, -19.2142)
  line L5816 (177.2861, -19.2142) -> (177.2861, -20.1558)
  line L5817 (179.5846, -20.1558) -> (179.5846, -19.2142)
  line L5818 (180.5962, -19.2142) -> (180.5962, -20.1558)
  line L5819 (180.5962, -20.1558) -> (179.5846, -20.1558)
  line L5820 (179.5846, -19.2142) -> (180.5962, -19.2142)
  line L5821 (177.2861, -77.3314) -> (176.2745, -77.3314)
  line L5822 (176.2745, -76.3898) -> (177.2861, -76.3898)
  line L5823 (176.2745, -77.3314) -> (176.2745, -76.3898)
  line L5824 (177.2861, -76.3898) -> (177.2861, -77.3314)
  line L5825 (180.5962, -76.3898) -> (180.5962, -77.3314)
  line L5826 (179.5846, -77.3314) -> (179.5846, -76.3898)
  line L5827 (179.5846, -76.3898) -> (180.5962, -76.3898)
  line L5828 (180.5962, -77.3314) -> (179.5846, -77.3314)
  line L5829 (176.2745, -57.327) -> (177.2861, -57.327)
  line L5830 (177.2861, -58.2686) -> (176.2745, -58.2686)
  line L5831 (176.2745, -58.2686) -> (176.2745, -57.327)
  line L5832 (177.2861, -57.327) -> (177.2861, -58.2686)
  line L5833 (179.5846, -58.2686) -> (179.5846, -57.327)
  line L5834 (179.5846, -57.327) -> (180.5962, -57.327)
  line L5835 (180.5962, -57.327) -> (180.5962, -58.2686)
  line L5836 (180.5962, -58.2686) -> (179.5846, -58.2686)
  line L5837 (177.2861, -38.2643) -> (177.2861, -39.2059)
  line L5838 (176.2745, -38.2643) -> (177.2861, -38.2643)
  line L5839 (176.2745, -39.2059) -> (176.2745, -38.2643)
  line L5840 (177.2861, -39.2059) -> (176.2745, -39.2059)
  line L5841 (180.5962, -39.2059) -> (179.5846, -39.2059)
  line L5842 (179.5846, -38.2643) -> (180.5962, -38.2643)
  line L5843 (179.5846, -39.2059) -> (179.5846, -38.2643)
  line L5844 (180.5962, -38.2643) -> (180.5962, -39.2059)
  line L5845 (101.0859, -76.3898) -> (101.0859, -77.3314)
  line L5846 (100.0743, -77.3314) -> (100.0743, -76.3898)
  line L5847 (101.0859, -77.3314) -> (100.0743, -77.3314)
  line L5848 (100.0743, -76.3898) -> (101.0859, -76.3898)
  line L5849 (103.3845, -76.3898) -> (104.3961, -76.3898)
  line L5850 (104.3961, -76.3898) -> (104.3961, -77.3314)
  line L5851 (103.3845, -77.3314) -> (103.3845, -76.3898)
  line L5852 (104.3961, -77.3314) -> (103.3845, -77.3314)
  line L5853 (101.0859, -58.2686) -> (100.0743, -58.2686)
  line L5854 (100.0743, -57.327) -> (101.0859, -57.327)
  line L5855 (100.0743, -58.2686) -> (100.0743, -57.327)
  line L5856 (101.0859, -57.327) -> (101.0859, -58.2686)
  line L5857 (103.3845, -57.327) -> (104.3961, -57.327)
  line L5858 (104.3961, -58.2686) -> (103.3845, -58.2686)
  line L5859 (104.3961, -57.327) -> (104.3961, -58.2686)
  line L5860 (103.3845, -58.2686) -> (103.3845, -57.327)
  line L5861 (100.0743, -20.1558) -> (100.0743, -19.2142)
  line L5862 (101.0859, -19.2142) -> (101.0859, -20.1558)
  line L5863 (100.0743, -19.2142) -> (101.0859, -19.2142)
  line L5864 (101.0859, -20.1558) -> (100.0743, -20.1558)
  line L5865 (103.3845, -20.1558) -> (103.3845, -19.2142)
  line L5866 (103.3845, -19.2142) -> (104.3961, -19.2142)
  line L5867 (104.3961, -19.2142) -> (104.3961, -20.1558)
  line L5868 (104.3961, -20.1558) -> (103.3845, -20.1558)
  line L5869 (101.0859, -39.2059) -> (100.0743, -39.2059)
  line L5870 (101.0859, -38.2643) -> (101.0859, -39.2059)
  line L5871 (100.0743, -39.2059) -> (100.0743, -38.2643)
  line L5872 (100.0743, -38.2643) -> (101.0859, -38.2643)
  line L5873 (103.3845, -39.2059) -> (103.3845, -38.2643)
  line L5874 (103.3845, -38.2643) -> (104.3961, -38.2643)
  line L5875 (104.3961, -38.2643) -> (104.3961, -39.2059)
  line L5876 (104.3961, -39.2059) -> (103.3845, -39.2059)
  line L5877 (119.1244, -19.2142) -> (120.136, -19.2142)
  line L5878 (120.136, -19.2142) -> (120.136, -20.1558)
  line L5879 (120.136, -20.1558) -> (119.1244, -20.1558)
  line L5880 (119.1244, -20.1558) -> (119.1244, -19.2142)
  line L5881 (122.4345, -19.2142) -> (123.4461, -19.2142)
  line L5882 (122.4345, -20.1558) -> (122.4345, -19.2142)
  line L5883 (123.4461, -19.2142) -> (123.4461, -20.1558)
  line L5884 (123.4461, -20.1558) -> (122.4345, -20.1558)
  line L5885 (120.136, -58.2686) -> (119.1244, -58.2686)
  line L5886 (119.1244, -58.2686) -> (119.1244, -57.327)
  line L5887 (120.136, -57.327) -> (120.136, -58.2686)
  line L5888 (119.1244, -57.327) -> (120.136, -57.327)
  line L5889 (123.4461, -58.2686) -> (122.4345, -58.2686)
  line L5890 (123.4461, -57.327) -> (123.4461, -58.2686)
  line L5891 (122.4345, -57.327) -> (123.4461, -57.327)
  line L5892 (122.4345, -58.2686) -> (122.4345, -57.327)
  line L5893 (119.1244, -39.2059) -> (119.1244, -38.2643)
  line L5894 (120.136, -38.2643) -> (120.136, -39.2059)
  line L5895 (120.136, -39.2059) -> (119.1244, -39.2059)
  line L5896 (119.1244, -38.2643) -> (120.136, -38.2643)
  line L5897 (123.4461, -39.2059) -> (122.4345, -39.2059)
  line L5898 (122.4345, -38.2643) -> (123.4461, -38.2643)
  line L5899 (122.4345, -39.2059) -> (122.4345, -38.2643)
  line L5900 (123.4461, -38.2643) -> (123.4461, -39.2059)
  line L5901 (119.1244, -76.3898) -> (120.136, -76.3898)
  line L5902 (119.1244, -77.3314) -> (119.1244, -76.3898)
  line L5903 (120.136, -77.3314) -> (119.1244, -77.3314)
  line L5904 (120.136, -76.3898) -> (120.136, -77.3314)
  line L5905 (122.4345, -76.3898) -> (123.4461, -76.3898)
  line L5906 (122.4345, -77.3314) -> (122.4345, -76.3898)
  line L5907 (123.4461, -76.3898) -> (123.4461, -77.3314)
  line L5908 (123.4461, -77.3314) -> (122.4345, -77.3314)
  line L5909 (4.8241, -76.3898) -> (5.8358, -76.3898)
  line L5910 (5.8358, -77.3314) -> (4.8241, -77.3314)
  line L5911 (4.8241, -77.3314) -> (4.8241, -76.3898)
  line L5912 (5.8358, -76.3898) -> (5.8358, -77.3314)
  line L5913 (8.1343, -77.3314) -> (8.1343, -76.3898)
  line L5914 (9.1459, -76.3898) -> (9.1459, -77.3314)
  line L5915 (9.1459, -77.3314) -> (8.1343, -77.3314)
  line L5916 (8.1343, -76.3898) -> (9.1459, -76.3898)
  line L5917 (24.8858, -76.3898) -> (24.8858, -77.3314)
  line L5918 (24.8858, -77.3314) -> (23.8742, -77.3314)
  line L5919 (23.8742, -76.3898) -> (24.8858, -76.3898)
  line L5920 (23.8742, -77.3314) -> (23.8742, -76.3898)
  line L5921 (28.1959, -76.3898) -> (28.1959, -77.3314)
  line L5922 (27.1843, -77.3314) -> (27.1843, -76.3898)
  line L5923 (27.1843, -76.3898) -> (28.1959, -76.3898)
  line L5924 (28.1959, -77.3314) -> (27.1843, -77.3314)
  line L5925 (42.9242, -77.3314) -> (42.9242, -76.3898)
  line L5926 (43.9358, -76.3898) -> (43.9358, -77.3314)
  line L5927 (43.9358, -77.3314) -> (42.9242, -77.3314)
  line L5928 (42.9242, -76.3898) -> (43.9358, -76.3898)
  line L5929 (46.2344, -76.3898) -> (47.246, -76.3898)
  line L5930 (47.246, -77.3314) -> (46.2344, -77.3314)
  line L5931 (47.246, -76.3898) -> (47.246, -77.3314)
  line L5932 (46.2344, -77.3314) -> (46.2344, -76.3898)
  line L5933 (62.9859, -19.2142) -> (62.9859, -20.1558)
  line L5934 (62.9859, -20.1558) -> (61.9743, -20.1558)
  line L5935 (61.9743, -20.1558) -> (61.9743, -19.2142)
  line L5936 (61.9743, -19.2142) -> (62.9859, -19.2142)
  line L5937 (66.296, -20.1558) -> (65.2844, -20.1558)
  line L5938 (66.296, -19.2142) -> (66.296, -20.1558)
  line L5939 (65.2844, -20.1558) -> (65.2844, -19.2142)
  line L5940 (65.2844, -19.2142) -> (66.296, -19.2142)
  line L5941 (61.9743, -76.3898) -> (62.9859, -76.3898)
  line L5942 (61.9743, -77.3314) -> (61.9743, -76.3898)
  line L5943 (62.9859, -77.3314) -> (61.9743, -77.3314)
  line L5944 (62.9859, -76.3898) -> (62.9859, -77.3314)
  line L5945 (65.2844, -77.3314) -> (65.2844, -76.3898)
  line L5946 (66.296, -77.3314) -> (65.2844, -77.3314)
  line L5947 (65.2844, -76.3898) -> (66.296, -76.3898)
  line L5948 (66.296, -76.3898) -> (66.296, -77.3314)
  line L5949 (61.9743, -38.2643) -> (62.9859, -38.2643)
  line L5950 (62.9859, -39.2059) -> (61.9743, -39.2059)
  line L5951 (62.9859, -38.2643) -> (62.9859, -39.2059)
  line L5952 (61.9743, -39.2059) -> (61.9743, -38.2643)
  line L5953 (66.296, -38.2643) -> (66.296, -39.2059)
  line L5954 (65.2844, -38.2643) -> (66.296, -38.2643)
  line L5955 (66.296, -39.2059) -> (65.2844, -39.2059)
  line L5956 (65.2844, -39.2059) -> (65.2844, -38.2643)
  line L5957 (61.9743, -57.327) -> (62.9859, -57.327)
  line L5958 (62.9859, -58.2686) -> (61.9743, -58.2686)
  line L5959 (62.9859, -57.327) -> (62.9859, -58.2686)
  line L5960 (61.9743, -58.2686) -> (61.9743, -57.327)
  line L5961 (65.2844, -58.2686) -> (65.2844, -57.327)
  line L5962 (66.296, -57.327) -> (66.296, -58.2686)
  line L5963 (65.2844, -57.327) -> (66.296, -57.327)
  line L5964 (66.296, -58.2686) -> (65.2844, -58.2686)
  line L5965 (82.0359, -39.2059) -> (81.0243, -39.2059)
  line L5966 (81.0243, -39.2059) -> (81.0243, -38.2643)
  line L5967 (81.0243, -38.2643) -> (82.0359, -38.2643)
  line L5968 (82.0359, -38.2643) -> (82.0359, -39.2059)
  line L5969 (85.346, -39.2059) -> (84.3344, -39.2059)
  line L5970 (85.346, -38.2643) -> (85.346, -39.2059)
  line L5971 (84.3344, -39.2059) -> (84.3344, -38.2643)
  line L5972 (84.3344, -38.2643) -> (85.346, -38.2643)
  line L5973 (81.0243, -77.3314) -> (81.0243, -76.3898)
  line L5974 (82.0359, -76.3898) -> (82.0359, -77.3314)
  line L5975 (82.0359, -77.3314) -> (81.0243, -77.3314)
  line L5976 (81.0243, -76.3898) -> (82.0359, -76.3898)
  line L5977 (84.3344, -77.3314) -> (84.3344, -76.3898)
  line L5978 (85.346, -76.3898) -> (85.346, -77.3314)
  line L5979 (84.3344, -76.3898) -> (85.346, -76.3898)
  line L5980 (85.346, -77.3314) -> (84.3344, -77.3314)
  line L5981 (82.0359, -20.1558) -> (81.0243, -20.1558)
  line L5982 (81.0243, -20.1558) -> (81.0243, -19.2142)
  line L5983 (81.0243, -19.2142) -> (82.0359, -19.2142)
  line L5984 (82.0359, -19.2142) -> (82.0359, -20.1558)
  line L5985 (85.346, -20.1558) -> (84.3344, -20.1558)
  line L5986 (84.3344, -19.2142) -> (85.346, -19.2142)
  line L5987 (85.346, -19.2142) -> (85.346, -20.1558)
  line L5988 (84.3344, -20.1558) -> (84.3344, -19.2142)
  line L5989 (82.0359, -57.327) -> (82.0359, -58.2686)
  line L5990 (81.0243, -58.2686) -> (81.0243, -57.327)
  line L5991 (82.0359, -58.2686) -> (81.0243, -58.2686)
  line L5992 (81.0243, -57.327) -> (82.0359, -57.327)
  line L5993 (84.3344, -57.327) -> (85.346, -57.327)
  line L5994 (84.3344, -58.2686) -> (84.3344, -57.327)
  line L5995 (85.346, -58.2686) -> (84.3344, -58.2686)
  line L5996 (85.346, -57.327) -> (85.346, -58.2686)
  line L5997 (4.8241, -58.2686) -> (4.8241, -57.327)
  line L5998 (5.8358, -57.327) -> (5.8358, -58.2686)
  line L5999 (4.8241, -57.327) -> (5.8358, -57.327)
  line L6000 (5.8358, -58.2686) -> (4.8241, -58.2686)
  line L6001 (9.1459, -57.327) -> (9.1459, -58.2686)
  line L6002 (8.1343, -57.327) -> (9.1459, -57.327)
  line L6003 (8.1343, -58.2686) -> (8.1343, -57.327)
  line L6004 (9.1459, -58.2686) -> (8.1343, -58.2686)
  line L6005 (5.8358, -20.1558) -> (4.8241, -20.1558)
  line L6006 (5.8358, -19.2142) -> (5.8358, -20.1558)
  line L6007 (4.8241, -20.1558) -> (4.8241, -19.2142)
  line L6008 (4.8241, -19.2142) -> (5.8358, -19.2142)
  line L6009 (8.1343, -19.2142) -> (9.1459, -19.2142)
  line L6010 (8.1343, -20.1558) -> (8.1343, -19.2142)
  line L6011 (9.1459, -19.2142) -> (9.1459, -20.1558)
  line L6012 (9.1459, -20.1558) -> (8.1343, -20.1558)
  line L6013 (5.8358, -39.2059) -> (4.8241, -39.2059)
  line L6014 (4.8241, -38.2643) -> (5.8358, -38.2643)
  line L6015 (4.8241, -39.2059) -> (4.8241, -38.2643)
  line L6016 (5.8358, -38.2643) -> (5.8358, -39.2059)
  line L6017 (8.1343, -39.2059) -> (8.1343, -38.2643)
  line L6018 (9.1459, -39.2059) -> (8.1343, -39.2059)
  line L6019 (9.1459, -38.2643) -> (9.1459, -39.2059)
  line L6020 (8.1343, -38.2643) -> (9.1459, -38.2643)
  line L6021 (23.8742, -39.2059) -> (23.8742, -38.2643)
  line L6022 (24.8858, -39.2059) -> (23.8742, -39.2059)
  line L6023 (23.8742, -38.2643) -> (24.8858, -38.2643)
  line L6024 (24.8858, -38.2643) -> (24.8858, -39.2059)
  line L6025 (28.1959, -39.2059) -> (27.1843, -39.2059)
  line L6026 (27.1843, -38.2643) -> (28.1959, -38.2643)
  line L6027 (27.1843, -39.2059) -> (27.1843, -38.2643)
  line L6028 (28.1959, -38.2643) -> (28.1959, -39.2059)
  line L6029 (23.8742, -19.2142) -> (24.8858, -19.2142)
  line L6030 (24.8858, -19.2142) -> (24.8858, -20.1558)
  line L6031 (24.8858, -20.1558) -> (23.8742, -20.1558)
  line L6032 (23.8742, -20.1558) -> (23.8742, -19.2142)
  line L6033 (27.1843, -20.1558) -> (27.1843, -19.2142)
  line L6034 (28.1959, -19.2142) -> (28.1959, -20.1558)
  line L6035 (28.1959, -20.1558) -> (27.1843, -20.1558)
  line L6036 (27.1843, -19.2142) -> (28.1959, -19.2142)
  line L6037 (24.8858, -57.327) -> (24.8858, -58.2686)
  line L6038 (24.8858, -58.2686) -> (23.8742, -58.2686)
  line L6039 (23.8742, -57.327) -> (24.8858, -57.327)
  line L6040 (23.8742, -58.2686) -> (23.8742, -57.327)
  line L6041 (27.1843, -57.327) -> (28.1959, -57.327)
  line L6042 (28.1959, -58.2686) -> (27.1843, -58.2686)
  line L6043 (27.1843, -58.2686) -> (27.1843, -57.327)
  line L6044 (28.1959, -57.327) -> (28.1959, -58.2686)
  line L6045 (43.9358, -19.2142) -> (43.9358, -20.1558)
  line L6046 (42.9242, -19.2142) -> (43.9358, -19.2142)
  line L6047 (43.9358, -20.1558) -> (42.9242, -20.1558)
  line L6048 (42.9242, -20.1558) -> (42.9242, -19.2142)
  line L6049 (46.2344, -20.1558) -> (46.2344, -19.2142)
  line L6050 (47.246, -19.2142) -> (47.246, -20.1558)
  line L6051 (46.2344, -19.2142) -> (47.246, -19.2142)
  line L6052 (47.246, -20.1558) -> (46.2344, -20.1558)
  line L6053 (43.9358, -57.327) -> (43.9358, -58.2686)
  line L6054 (42.9242, -58.2686) -> (42.9242, -57.327)
  line L6055 (42.9242, -57.327) -> (43.9358, -57.327)
  line L6056 (43.9358, -58.2686) -> (42.9242, -58.2686)
  line L6057 (47.246, -58.2686) -> (46.2344, -58.2686)
  line L6058 (46.2344, -58.2686) -> (46.2344, -57.327)
  line L6059 (46.2344, -57.327) -> (47.246, -57.327)
  line L6060 (47.246, -57.327) -> (47.246, -58.2686)
  line L6061 (43.9358, -39.2059) -> (42.9242, -39.2059)
  line L6062 (42.9242, -39.2059) -> (42.9242, -38.2643)
  line L6063 (43.9358, -38.2643) -> (43.9358, -39.2059)
  line L6064 (42.9242, -38.2643) -> (43.9358, -38.2643)
  line L6065 (47.246, -39.2059) -> (46.2344, -39.2059)
  line L6066 (47.246, -38.2643) -> (47.246, -39.2059)
  line L6067 (46.2344, -38.2643) -> (47.246, -38.2643)
  line L6068 (46.2344, -39.2059) -> (46.2344, -38.2643)
  line L6069 (215.3862, -20.1558) -> (214.3746, -20.1558)
  line L6070 (215.3862, -19.2142) -> (215.3862, -20.1558)
  line L6071 (214.3746, -19.2142) -> (215.3862, -19.2142)
  line L6072 (214.3746, -20.1558) -> (214.3746, -19.2142)
  line L6073 (217.6847, -20.1558) -> (217.6847, -19.2142)
  line L6074 (217.6847, -19.2142) -> (218.6963, -19.2142)
  line L6075 (218.6963, -20.1558) -> (217.6847, -20.1558)
  line L6076 (218.6963, -19.2142) -> (218.6963, -20.1558)
  line L6077 (215.3862, -77.3314) -> (214.3746, -77.3314)
  line L6078 (214.3746, -76.3898) -> (215.3862, -76.3898)
  line L6079 (214.3746, -77.3314) -> (214.3746, -76.3898)
  line L6080 (215.3862, -76.3898) -> (215.3862, -77.3314)
  line L6081 (218.6963, -77.3314) -> (217.6847, -77.3314)
  line L6082 (217.6847, -76.3898) -> (218.6963, -76.3898)
  line L6083 (217.6847, -77.3314) -> (217.6847, -76.3898)
  line L6084 (218.6963, -76.3898) -> (218.6963, -77.3314)
  line L6085 (214.3746, -58.2686) -> (214.3746, -57.327)
  line L6086 (214.3746, -57.327) -> (215.3862, -57.327)
  line L6087 (215.3862, -58.2686) -> (214.3746, -58.2686)
  line L6088 (215.3862, -57.327) -> (215.3862, -58.2686)
  line L6089 (217.6847, -57.327) -> (218.6963, -57.327)
  line L6090 (218.6963, -57.327) -> (218.6963, -58.2686)
  line L6091 (217.6847, -58.2686) -> (217.6847, -57.327)
  line L6092 (218.6963, -58.2686) -> (217.6847, -58.2686)
  line L6093 (215.3862, -39.2059) -> (214.3746, -39.2059)
  line L6094 (214.3746, -38.2643) -> (215.3862, -38.2643)
  line L6095 (214.3746, -39.2059) -> (214.3746, -38.2643)
  line L6096 (215.3862, -38.2643) -> (215.3862, -39.2059)
  line L6097 (217.6847, -39.2059) -> (217.6847, -38.2643)
  line L6098 (218.6963, -38.2643) -> (218.6963, -39.2059)
  line L6099 (217.6847, -38.2643) -> (218.6963, -38.2643)
  line L6100 (218.6963, -39.2059) -> (217.6847, -39.2059)
  line L6101 (196.3361, -38.2643) -> (196.3361, -39.2059)
  line L6102 (195.3245, -39.2059) -> (195.3245, -38.2643)
  line L6103 (196.3361, -39.2059) -> (195.3245, -39.2059)
  line L6104 (195.3245, -38.2643) -> (196.3361, -38.2643)
  line L6105 (198.6347, -39.2059) -> (198.6347, -38.2643)
  line L6106 (199.6463, -38.2643) -> (199.6463, -39.2059)
  line L6107 (199.6463, -39.2059) -> (198.6347, -39.2059)
  line L6108 (198.6347, -38.2643) -> (199.6463, -38.2643)
  line L6109 (195.3245, -77.3314) -> (195.3245, -76.3898)
  line L6110 (196.3361, -77.3314) -> (195.3245, -77.3314)
  line L6111 (196.3361, -76.3898) -> (196.3361, -77.3314)
  line L6112 (195.3245, -76.3898) -> (196.3361, -76.3898)